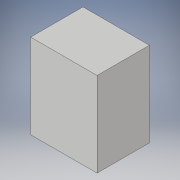
# Autodesk Inventor part: BlockShooter
Saved by Autodesk Inventor 2019 (Build 230136000, 136)
## iProperties
Created: 2020-01-25
Part Number: BlockShooter
Material: Generic
Document SubType Name: Modeling
Designer: james
Density: 1 g/cm^3
Appearance: Default
Author: james
Autodesk Inventor part; units mm, degrees
ref_plane "YZ Plane" through (0, 0, 0) normal (1, 0, 0) x (0, 1, 0)
ref_plane "XZ Plane" through (0, 0, 0) normal (0, 1, 0) x (-1, 0, 0)
ref_plane "XY Plane" through (0, 0, 0) normal (0, 0, 1) x (1, 0, 0)
sketch "Sketch1" plane through (0, 0, 0) normal (1, 0, 0) x (0, 1, 0)
  line L0 (190.5544, 164.3929) -> (-342.8456, 164.3929)
  line L1 (-342.8456, 164.3929) -> (-342.8456, -165.8071)
  line L2 (-342.8456, -165.8071) -> (190.5544, -165.8071)
  line L3 (190.5544, -165.8071) -> (190.5544, 164.3929)
  point P0 (0, 0)
  dimension "d0" = 330.2
  dimension "d1" = 533.4
  constraints: 8 end point, 2 parallel, 1 horizontal, 1 perpendicular
  measures "d0" distance of L2.end L0.start
  measures "d1" distance of L0.start L0.end
extrude "Extrusion1" add sketch "Sketch1" along normal blind 419.1
body "Solid1"
